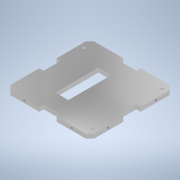
# Autodesk Inventor part: stackframesupport
Saved by Autodesk Inventor 2022 (Build 260153000, 153)
## iProperties
Created: 2022-02-12
Part Number: stackframesupport
Material: Aluminum 6061
Document SubType Name: Modeling
Designer: Bowen
Density: 2.7 g/cm^3
Appearance: Aluminum - Flat
Author: Bowen
Autodesk Inventor part; units mm, degrees
ref_plane "YZ Plane" through (0, 0, 0) normal (1, 0, 0) x (0, 1, 0)
ref_plane "XZ Plane" through (0, 0, 0) normal (0, 1, 0) x (-1, 0, 0)
ref_plane "XY Plane" through (0, 0, 0) normal (0, 0, 1) x (1, 0, 0)
sketch "Sketch1" plane through (0, 0, 0) normal (0, 1, 0) x (-1, 0, 0)
  line L0 (48.5, 48.5) -> (-48.5, 48.5)
  line L1 (-48.5, 48.5) -> (-48.5, -48.5)
  line L2 (-48.5, -48.5) -> (48.5, -48.5)
  line L3 (48.5, -48.5) -> (48.5, 48.5)
  point P0 (0, 0)
  point P1 (48.5, 0)
  point P2 (0, -48.5)
  dimension "d0" = 97
  dimension "d1" = 97
  constraints: 8 end point, 2 midpoint, 2 parallel, 1 horizontal, 1 horizontal alignment, 1 perpendicular, 1 vertical alignment
  measures "d0" distance of L1.end L2.end
  measures "d1" distance of L2.end L0.start
extrude "Extrusion1" add sketch "Sketch1" along normal mid plane 5
sketch "Sketch2" plane through (0, -2.5, 0) normal (0, -1, 0) x (1, 0, 0)
  line L0 (-42.865, 37.465) -> (-42.865, -36.195) construction
  line L1 (42.865, 40.005) -> (42.865, -40.005) construction
  line L2 (-42.865, 6.4948) -> (42.865, 6.4948) construction
  point P0 (0, 0)
  point P1 (42.865, 0)
  point P2 (0, 6.4948)
  dimension "d4" = 73.66
  dimension "d5" = 80.01
  dimension "d6" = 85.73
  dimension "d7" = 3.81
  constraints: 6 end point, 3 vertical alignment, 2 midpoint, 2 point on line, 2 vertical, 1 horizontal alignment, 1 perpendicular
  measures "d4" distance of L0.start L0.end
  measures "d5" distance of L1.end L1.start
  measures "d6" horizontal distance of L1.end L0.end
  measures "d7" vertical distance of L1.end L0.end
hole "Hole1" at (-42.865, -2.5, 37.465) at (42.865, -2.5, 40.005) at (-42.865, -2.5, -36.195) at (42.865, -2.5, -40.005) direction (0, 1, 0) diameter 3.6 end through all clearance for "Flat Head Machine Screw" size "M3" standard "Ansi Metric M Profile"
chamfer "Chamfer1" distance 5 angle 45 4 edges at (48.5, 0, -48.5) (-48.5, 0, -48.5) (48.5, 0, 48.5) (-48.5, 0, 48.5)
sketch "Sketch3" plane through (48.5, -2.5, 43.5) normal (1, 0, 0) x (0, 0, -1)
  point P0 (43.5, 2.5)
  point P1 (71, 2.5)
  point P2 (16, 2.5)
  dimension "d18" = 55
  dimension "d19" = 27.5
  constraints: 2 horizontal alignment
  measures "d18" distance of point (16, 2.5) point (71, 2.5)
  measures "d19" distance of point (16, 2.5) point (43.5, 2.5)
hole "Hole2" at (48.5, 0, -27.5) at (48.5, 0, 27.5) direction (-1, 0, 0) diameter 2.1565 depth 4 thread size "4-40 UNC" class "2B" standard "ANSI Unified Screw Threads"
pattern_circular "Circular Pattern1" count 4 over 360 about axis through (0, -10, 0) along (0, 1, 0) of "Hole2"
sketch "Sketch5" plane through (0, 2.5, 0) normal (0, 1, 0) x (1, 0, 0)
  line L0 (-15, 25) -> (0, 25)
  line L1 (0, 25) -> (0, -25)
  line L2 (0, -25) -> (-15, -25)
  line L3 (-15, -25) -> (-15, 25)
  point P0 (0, 0)
  point P1 (0, 0)
  dimension "d38" = 15
  dimension "d39" = 50
  constraints: 8 end point, 2 parallel, 1 coincident, 1 horizontal, 1 midpoint, 1 perpendicular
  measures "d38" distance of L0.start L0.end
  measures "d39" distance of L2.end L0.start
extrude "Extrusion3" cut sketch "Sketch5" against normal through all
sketch "Sketch6" plane through (0, 2.5, 0) normal (0, 1, 0) x (1, 0, 0)
  line L0 (-48.5, 43.5) -> (-48.5, -43.5) projected
  line L1 (-43.5, 10) -> (-48.5, 10)
  line L2 (-48.5, 10) -> (-48.5, -10)
  line L3 (-48.5, -10) -> (-43.5, -10)
  line L4 (-43.5, -10) -> (-43.5, 10)
  point P0 (0, 0)
  point P1 (-48.5, 0)
  dimension "d42" = 5
  dimension "d43" = 20
  constraints: 8 end point, 2 midpoint, 2 parallel, 1 horizontal, 1 perpendicular, 1 point on line
  measures "d42" distance of L2.end L3.end
  measures "d43" distance of L3.end L1.start
extrude "Extrusion4" cut sketch "Sketch6" against normal through all
pattern_circular "Circular Pattern3" count 4 over 360 about axis through (0, -10, 0) along (0, 1, 0) of "Extrusion4"
equation "\"d1\" = d0"
equation "\"d19\" = 0.5 * d18"
body "Solid1"
